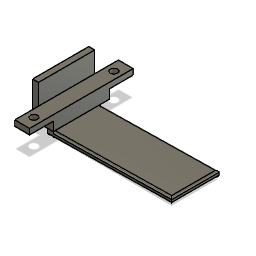
clip (Autodesk Fusion 360 design; units mm, degrees)
Autodesk Fusion 360 part; units mm, degrees
sketch "Sketch1" plane through (0, 0, 0) normal (0, 1, 0) x (1, 0, 0)
  line L0 (0, 0) -> (7, 0)
  line L1 (7, 0) -> (7, -19)
  line L2 (7, -19) -> (0, -19)
  line L3 (0, -19) -> (0, 0)
  dimension "d1" = 7
  dimension "d2" = 19
  constraint horizontal L0
  constraint vertical L1
  constraint horizontal L2
  constraint vertical L3
  constraint coincident L0.start L3.end
  measures "d1" distance of L0.start L0.end
  measures "d2" distance of L0.start L2.end
extrude "Extrude1" add sketch "Sketch1" along normal blind 4.95
sketch "Sketch3" plane through (0, 4.95, 0) normal (0, 1, 0) x (-1, 0, 0)
  line L0 (0, 19) -> (-7, 19)
  line L1 (-7, 19) -> (-7, 0)
  line L2 (-7, 0) -> (0, 0)
  line L3 (0, 0) -> (0, 19)
  line L4 (0, 0) -> (-2, 0)
  line L5 (-2, 0) -> (-2, 19)
  line L6 (-2, 19) -> (0, 19)
  line L7 (0, 19) -> (0, 0)
  dimension "d8" = 2
  constraint horizontal L4
  constraint vertical L5
  constraint horizontal L6
  constraint vertical L7
  constraint coincident L0 L5.end
  constraint coincident L2.end L3.start
  measures "d8" distance of L5.end L0.start
extrude "Extrude3" add sketch "Sketch3" along normal blind 6.95 contours L0 L2 L3 L4 L5 L6 L7
ref_plane "WorkPlane1" through (3.5, 5.95, 9.5) normal (0, 0, 1) x (1, 0, 0)
sketch "Sketch4" plane through (0, 0, 19) normal (0, 0, 1) x (1, 0, 0)
  line L0 (0, 0) -> (7, 0)
  line L1 (7, 0) -> (7, 4.95)
  line L2 (7, 4.95) -> (2, 4.95)
  line L3 (2, 4.95) -> (2, 11.9)
  line L4 (2, 11.9) -> (0, 11.9)
  line L5 (0, 11.9) -> (0, 0)
  line L6 (2, 4.95) -> (7, 4.95)
  line L7 (7, 4.95) -> (7, 3.05)
  line L8 (7, 3.05) -> (2, 3.05)
  line L9 (2, 3.05) -> (2, 4.95)
  dimension "d21" = 3.05
  constraint horizontal L6
  constraint vertical L7
  constraint horizontal L8
  constraint vertical L9
  constraint coincident L2.end L3.start
  constraint coincident L1 L7.end
  measures "d21" distance of L0 L8
extrude "Extrude4" add sketch "Sketch4" along normal blind 8 contours L1 L2 L6 L7 L8 L9
mirror "Mirror1" about plane through (3.5, 5.95, 9.5) normal (0, 0, 1) of "Extrude4"
sketch "Sketch5" plane through (0, 4.95, 0) normal (0, 1, 0) x (-1, 0, 0)
  line L0 (-7, 27) -> (-7, -8)
  line L1 (-7, -8) -> (-2, -8)
  line L2 (-2, -8) -> (-2, 0)
  line L3 (-2, 0) -> (-2, 19)
  line L4 (-2, 19) -> (-2, 27)
  line L5 (-2, 27) -> (-7, 27)
  line L6 (0, 19) -> (-2, 19)
  line L7 (0.7, 9.5) -> (-7.7, 9.5)
  point P0 (-4.5, 23)
  point P1 (-4.5, -4)
  dimension "d14" = 2.5
  dimension "d15" = 2.5
  dimension "d16" = 4
  dimension "d17" = 5
  constraint symmetric P0 L7 P1
  measures "d14" distance of L4 P0
  measures "d15" distance of L0 P0
  measures "d16" distance of L5 P0
hole "Hole1" at (4.5, 4.95, -4) at (4.5, 4.95, 23) direction (0, -1, 0) diameter 2.4 depth 2 tip angle 118
sketch "Sketch6" plane through (0, 0, 0) normal (0, -1, 0) x (1, 0, 0)
  line L0 (0, 0) -> (7, 0)
  line L1 (7, 0) -> (7, 19)
  line L2 (7, 19) -> (0, 19)
  line L3 (0, 19) -> (0, 0)
  line L4 (3.5, 17.5) -> (5.5, 17.5)
  line L5 (5.5, 17.5) -> (5.5, 1.5)
  line L6 (5.5, 1.5) -> (3.5, 1.5)
  line L7 (3.5, 1.5) -> (3.5, 17.5)
  dimension "d22" = 2
  dimension "d23" = 1.5
  dimension "d24" = 1.5
  dimension "d25" = 1.5
  constraint horizontal L4
  constraint vertical L5
  constraint horizontal L6
  constraint vertical L7
  measures "d22" distance of L4.start L4.end
  measures "d23" distance of L1 L5
  measures "d24" distance of L2 L4
  measures "d25" distance of L0 L6
extrude "Extrude5" add sketch "Sketch6" along normal blind 3.5 contours L4 L5 L6 L7
sketch "Sketch7" plane through (5.5, 0, 0) normal (1, 0, 0) x (0, 0, -1)
  line L0 (-1.5, 0) -> (-17.5, 0)
  line L1 (-17.5, 0) -> (-17.5, -3.5)
  line L2 (-17.5, -3.5) -> (-1.5, -3.5)
  line L3 (-1.5, -3.5) -> (-1.5, 0)
  line L4 (-17.5, -3.5) -> (-1.5, -3.5)
  line L5 (-1.5, -3.5) -> (-1.5, -1.5)
  line L6 (-1.5, -1.5) -> (-17.5, -1.5)
  line L7 (-17.5, -1.5) -> (-17.5, -3.5)
  dimension "d28" = 2
  constraint horizontal L4
  constraint vertical L5
  constraint horizontal L6
  constraint vertical L7
  constraint coincident L3 L5.end
  constraint coincident L1.end L2.start
  measures "d28" distance of L1.end L6.end
sketch "Sketch8" plane through (0, 0, 0) normal (0, 0, 1) x (1, 0, 0)
  line L0 (5.5, -3.6158) -> (45.5, -2.9158)
  line L1 (5.5, -3.5) -> (5.5, -1.5)
  dimension "d29" = 0.7
  dimension "d30" = 40
  constraint coincident L0.start L1
  measures "d29" vertical distance of L0.start L0.end
  measures "d30" horizontal distance of L0.start L0.end
sweep "Sweep1" add profiles "Sketch7" path "Sketch8" along L0 section 1 contours L1 L2 L3 L4 L5 L6 L7
fillet "Fillet1" radius 1 3 edges at (3.5, 0, 9.5) (4.5, 0, 1.5) (4.5, 0, 17.5)
fillet "Fillet1" radius 1 1 edges at (5.5, 0, 9.5)
fillet "Fillet2" radius 0.6 9 edges at (3.5, -3.5, 9.5) (25.5, -3.15, 1.5) (4.5, -3.5, 1.5) (4.5, -3.5, 17.5) (25.5, -3.15, 17.5) (45.5, -2.8, 9.5) (25.5, -1.15, 1.5) (25.5, -1.15, 17.5) (45.5, -0.8, 9.5)
